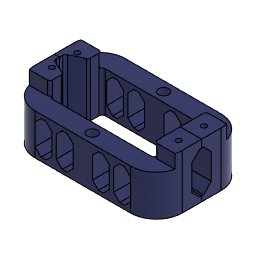
Servo Bracket v4 (Autodesk Fusion 360 design; units mm, degrees)
Autodesk Fusion 360 part; units mm, degrees
sketch "Sketch1" plane through (0, 0, 0) normal (0, 0, 1) x (1, 0, 0)
  line L0 (-28.5, 0) -> (28.5, 0)
  line L1 (28.5, 0) -> (28.5, -17.5)
  line L2 (28.5, -17.5) -> (-28.5, -17.5)
  line L3 (-28.5, -17.5) -> (-28.5, 0)
  line L4 (-20.2, 0) -> (20.2, 0)
  line L5 (20.2, 0) -> (20.2, -9)
  line L6 (19, -10.2) -> (-19, -10.2)
  line L7 (-20.2, -9) -> (-20.2, 0)
  arc A0 (-20.2, -9) -> (-19, -10.2) centre (-19, -9) ccw
  arc A1 (19, -10.2) -> (20.2, -9) centre (19, -9) ccw
  line L8 (-26.5, 0) -> (-26.5, -1.2659)
  line L9 (-25.7783, -2.3988) -> (-20.2, -5)
  arc A2 (-26.5, -1.2659) -> (-25.7783, -2.3988) centre (-25.25, -1.2659) ccw
  circle A3 centre (-24.5, -4.902) radius 1
  circle A4 centre (0, -13.85) radius 2
  line L10 (0, 0) -> (0, -20.883) construction
  circle A5 centre (24.5, -4.902) radius 1
  point P0 (20.2, -10.2)
  point P1 (-20.2, -10.2)
  dimension "d1" = 17.5
  dimension "d2" = 57
  dimension "d3" = 28.5
  dimension "d10" = 10.2
  dimension "d11" = 40.4
  dimension "d12" = 20.2
  dimension "d13" = 1.2
  dimension "d14" = 1.2
  dimension "d17" = 1.25
  dimension "d18" = 2
  dimension "d19" = 5
  dimension "d20" = 65
  dimension "d23" = 4.902
  dimension "d24" = 2
  dimension "d25" = 4
  dimension "d27" = 4
  dimension "d28" = 3.65
  dimension "d29" = 4
  dimension "d30" = 4.902
  constraint horizontal L0
  constraint vertical L1
  constraint horizontal L2
  constraint vertical L3
  constraint coincident L10.start L0
  constraint horizontal L4
  constraint vertical L5
  constraint horizontal L6
  constraint vertical L7
  constraint coincident L0 L4.start
  constraint coincident P1 L7
  constraint coincident P1 L6
  constraint tangent L7 A0
  constraint tangent L6 A0
  constraint coincident P0 L6
  constraint coincident P0 L5
  constraint tangent L6 A1
  constraint tangent L5 A1
  constraint coincident L0 L8.start
  constraint perpendicular L0 L8
  constraint coincident L7 L9.end
  constraint tangent L8 A2
  constraint tangent L9 A2
  constraint coincident L10.start origin
  constraint perpendicular L2 L10
  constraint coincident A4.centre L10
  constraint equal A3 A5
  measures "d1" distance of L0.start L2.end
  measures "d2" distance of L1.end L2.end
  measures "d3" distance of L10.start L1
  measures "d10" distance of L4.start P1
  measures "d11" distance of P0 P1
  measures "d12" distance of L10.start L7
  measures "d13" radius of A0
  measures "d14" radius of A1
  measures "d17" radius of A2
  measures "d18" distance of L3 L8
  measures "d19" distance of L0 L9.end
  measures "d20" angle of L7 L9
  measures "d23" distance of L0 A3.centre
  measures "d24" diameter of A3
  measures "d25" distance of L3 A3.centre
  measures "d27" diameter of A4
  measures "d28" distance of L2 A4.centre
  measures "d29" distance of L1 A5.centre
  measures "d30" distance of L0 A5.centre
extrude "Extrude1" add sketch "Sketch1" along normal blind 21 contours L0 L1 L2 L3 L5 L6 L7 A0 A1 L8 L9 A2 makes body 1
fillet "Fillet1" radius 10 2 edges at (-28.5, -17.5, 10.5) (28.5, -17.5, 10.5) on bodies 1
fillet "Fillet2" radius 1 1 edges at (-20.2, -5, 10.5) on bodies 1
sketch "Sketch3" plane through (0, 0, 21) normal (0, 0, 1) x (-1, 0, 0)
  arc A0 (20.2, 5.6371) -> (20.7774, 4.7308) centre (21.2, 5.6371) ccw
  line L0 (20.7774, 4.7308) -> (25.7783, 2.3988)
  arc A1 (26.5, 1.2659) -> (25.7783, 2.3988) centre (25.25, 1.2659) ccw
  line L1 (26.5, 1.2659) -> (26.5, 0)
  line L2 (26.5, 0) -> (28.5, 0)
  line L3 (28.5, 0) -> (28.5, 7.5)
  arc A2 (28.5, 7.5) -> (18.5, 17.5) centre (18.5, 7.5) ccw
  line L4 (18.5, 17.5) -> (-18.5, 17.5)
  arc A3 (-18.5, 17.5) -> (-28.5, 7.5) centre (-18.5, 7.5) ccw
  line L5 (-28.5, 7.5) -> (-28.5, 0)
  line L6 (-28.5, 0) -> (-20.2, 0)
  line L7 (-20.2, 0) -> (-20.2, 9)
  arc A4 (-19, 10.2) -> (-20.2, 9) centre (-19, 9) ccw
  line L8 (-19, 10.2) -> (19, 10.2)
  arc A5 (20.2, 9) -> (19, 10.2) centre (19, 9) ccw
  line L9 (20.2, 9) -> (20.2, 5.6371)
  circle A6 centre (24.5, 4.902) radius 1
  circle A7 centre (-24.5, 4.902) radius 1
  circle A8 centre (0, 13.85) radius 2
  line L10 (32.5, 10) -> (-32.5, 10)
  line L11 (-32.5, 10) -> (-32.5, 20)
  line L12 (-32.5, 20) -> (32.5, 20)
  line L13 (32.5, 20) -> (32.5, 10)
  dimension "d31" = 10
  dimension "d32" = 10
  dimension "d33" = 65
  dimension "d34" = 4
  constraint horizontal L10
  constraint vertical L11
  constraint horizontal L12
  constraint vertical L13
  measures "d31" distance of L6 L10
  measures "d32" distance of L10.end L11.end
  measures "d33" distance of L11.end L12.end
  measures "d34" distance of L5 L11
extrude "Extrude3" cut sketch "Sketch3" against normal blind 5.25 contours A2 L4 A3 A4 L8 A5 L10 | A2 L4 A3 L10 L11 L12 L13 bodies 1
fillet "Fillet3" radius 1 tangency weight 0.84674 2 edges at (-19.6633, -10, 18.375) (19.6633, -10, 18.375) on bodies 1
sketch "Sketch4" plane through (0, -17.5, 0) normal (0, -1, 0) x (1, 0, 0)
  line L0 (18.5, 15.75) -> (-18.5, 15.75)
  line L1 (-18.5, 15.75) -> (-18.5, 0)
  line L2 (-18.5, 0) -> (18.5, 0)
  line L3 (18.5, 0) -> (18.5, 15.75)
  line L4 (-10.25, 14.35) -> (-3.75, 14.35)
  line L5 (-3.75, 14.35) -> (-3.75, 1.4)
  line L6 (-3.75, 1.4) -> (-10.25, 1.4)
  line L7 (-10.25, 1.4) -> (-10.25, 14.35)
  line L8 (0, 0) -> (0, 19.5857) construction
  line L9 (-18.45, 14.35) -> (-11.95, 14.35)
  line L10 (-11.95, 14.35) -> (-11.95, 1.4)
  line L11 (-11.95, 1.4) -> (-18.45, 1.4)
  line L12 (-18.45, 1.4) -> (-18.45, 14.35)
  line L13 (2, 15.75) -> (-2, 15.75)
  line L14 (-2, 0) -> (2, 0)
  line L15 (-20.2, 0) -> (-20.2, 21)
  line L16 (-20.2, 21) -> (-20.2, 15.75)
  line L17 (-20.2, 15.75) -> (-20.2, 0)
  line L18 (3.75, 14.35) -> (3.75, 1.4)
  line L19 (11.95, 14.35) -> (11.95, 1.4)
  line L20 (3.75, 1.4) -> (10.25, 1.4)
  line L21 (11.95, 1.4) -> (18.45, 1.4)
  line L22 (10.25, 1.4) -> (10.25, 14.35)
  line L23 (10.25, 14.35) -> (3.75, 14.35)
  line L24 (18.45, 1.4) -> (18.45, 14.35)
  line L25 (18.45, 14.35) -> (11.95, 14.35)
  point P0 (18.5, 15.75)
  dimension "d40" = 1.4
  dimension "d41" = 1.4
  dimension "d42" = 6.5
  dimension "d44" = 1.75
  dimension "d45" = 1.75
  constraint horizontal L4
  constraint vertical L5
  constraint horizontal L6
  constraint vertical L7
  constraint coincident L8.start origin
  constraint perpendicular L0 L8
  constraint horizontal L9
  constraint vertical L10
  constraint horizontal L11
  constraint vertical L12
  constraint equal L4 L9
  constraint equal L7 L10
  constraint horizontal L4.start L9.end
  constraint symmetric L0.end L8 P0
  constraint symmetric L4.start L8 L22.end
  constraint symmetric L4.end L8 L18.start
  constraint symmetric L5.end L8 L18.end
  constraint symmetric L6.end L8 L20.end
  constraint symmetric L8 L9.start L24.end
  constraint symmetric L8 L9.end L19.start
  constraint symmetric L8 L10.end L19.end
  constraint symmetric L8 L11.end L21.end
  measures "d40" distance of L0 L4
  measures "d41" distance of L2 L6
  measures "d42" distance of L5.end L6.end
  measures "d44" distance of L5 L14.start
  measures "d45" distance of L12 L15
extrude "Extrude4" cut sketch "Sketch4" against normal through all contours L4 L5 L6 L7 | L9 L10 L11 L12 | L18 L20 L22 L23 | L19 L21 L24 L25 bodies 1
chamfer "Chamfer1" distance 2.3 angle 45 16 edges at (-18.45, -13.85, 14.35) (-10.25, -13.85, 14.35) (3.75, -13.85, 14.35) (11.95, -13.85, 14.35) (-11.95, -13.85, 14.35) (-3.75, -13.85, 14.35) (10.25, -13.85, 14.35) (18.45, -13.85, 14.35) (18.45, -13.85, 1.4) (10.25, -13.85, 1.4) (-3.75, -13.85, 1.4) (-11.95, -13.85, 1.4) (-18.45, -13.85, 1.4) (-10.25, -13.85, 1.4) (3.75, -13.85, 1.4) (11.95, -13.85, 1.4) on bodies 1
mirror "Mirror1" about plane through (0, 0, 0) normal (0, 1, 0) of bodies 1 makes body 2
sketch "Sketch5" plane through (28.5, 0, 0) normal (1, 0, 0) x (0, 1, 0)
  line L0 (-7.5, 21) -> (-7.5, 0)
  line L1 (-7.5, 0) -> (0, 0)
  line L2 (0, 0) -> (0, 21)
  line L3 (0, 21) -> (-7.5, 21)
  line L4 (-3.75, 18) -> (3.75, 18)
  line L5 (3.75, 18) -> (3.75, 2)
  line L6 (3.75, 2) -> (-3.75, 2)
  line L7 (-3.75, 2) -> (-3.75, 18)
  line L8 (0, 0) -> (0, 25.4329) construction
  line L9 (7.5, 21) -> (0, 21)
  dimension "d50" = 16
  dimension "d51" = 3
  dimension "d52" = 7.5
  constraint horizontal L4
  constraint vertical L5
  constraint horizontal L6
  constraint vertical L7
  constraint coincident L1.end L2.start
  constraint perpendicular L3 L8
  constraint symmetric L5 L7 L8
  measures "d50" distance of L4.end L5.end
  measures "d51" distance of L4 L9
  measures "d52" distance of L4.start L4.end
extrude "Extrude5" cut sketch "Sketch5" against normal blind 14 contours L2 L4 L5 L6 | L2 L4 L6 L7 bodies 1 2
chamfer "Chamfer2" distance 3 angle 45 4 edges at (24.35, 3.75, 2) (24.35, 3.75, 18) (24.35, -3.75, 2) (24.35, -3.75, 18) on bodies 1 2
equation "d3 = d2 / 2"
equation "d12 = d11 / 2"
equation "d23 = ( 9.804 / 2 ) * 1 mm"
equation "d28 = ( 7.3 / 2 ) * 1 mm"
equation "d30 = d23"
equation "d45 = d44"
